Autodesk Fusion 360 part; units mm, degrees
(part 3 of 12)
  arc A1088 (217.4364, 35.2653) -> (218.9364, 35.2653) centre (218.1864, 35.2653) ccw
  arc A1089 (218.9364, 35.2653) -> (217.4364, 35.2653) centre (218.1864, 35.2653) ccw
  arc A1090 (218.9364, 37.8053) -> (217.4364, 37.8053) centre (218.1864, 37.8053) ccw
  arc A1091 (217.4364, 37.8053) -> (218.9364, 37.8053) centre (218.1864, 37.8053) ccw
  arc A1092 (217.4364, 37.8053) -> (218.9364, 37.8053) centre (218.1864, 37.8053) ccw
  arc A1093 (218.9364, 37.8053) -> (217.4364, 37.8053) centre (218.1864, 37.8053) ccw
  arc A1094 (218.9364, 37.8053) -> (217.4364, 37.8053) centre (218.1864, 37.8053) ccw
  arc A1095 (217.4364, 37.8053) -> (218.9364, 37.8053) centre (218.1864, 37.8053) ccw
  arc A1096 (209.8164, 4.7852) -> (211.3164, 4.7852) centre (210.5664, 4.7852) ccw
  arc A1097 (211.3164, 4.7852) -> (209.8164, 4.7852) centre (210.5664, 4.7852) ccw
  arc A1098 (209.8164, 4.7852) -> (211.3164, 4.7852) centre (210.5664, 4.7852) ccw
  arc A1099 (211.3164, 4.7852) -> (209.8164, 4.7852) centre (210.5664, 4.7852) ccw
  arc A1100 (211.3164, 4.7852) -> (209.8164, 4.7852) centre (210.5664, 4.7852) ccw
  arc A1101 (209.8164, 4.7852) -> (211.3164, 4.7852) centre (210.5664, 4.7852) ccw
  arc A1102 (209.8164, 7.3252) -> (211.3164, 7.3252) centre (210.5664, 7.3252) ccw
  arc A1103 (211.3164, 7.3252) -> (209.8164, 7.3252) centre (210.5664, 7.3252) ccw
  arc A1104 (209.8164, 7.3252) -> (211.3164, 7.3252) centre (210.5664, 7.3252) ccw
  arc A1105 (211.3164, 7.3252) -> (209.8164, 7.3252) centre (210.5664, 7.3252) ccw
  arc A1106 (211.3164, 7.3252) -> (209.8164, 7.3252) centre (210.5664, 7.3252) ccw
  arc A1107 (209.8164, 7.3252) -> (211.3164, 7.3252) centre (210.5664, 7.3252) ccw
  arc A1108 (209.8164, 9.8652) -> (211.3164, 9.8652) centre (210.5664, 9.8652) ccw
  arc A1109 (211.3164, 9.8652) -> (209.8164, 9.8652) centre (210.5664, 9.8652) ccw
  arc A1110 (209.8164, 9.8652) -> (211.3164, 9.8652) centre (210.5664, 9.8652) ccw
  arc A1111 (211.3164, 9.8652) -> (209.8164, 9.8652) centre (210.5664, 9.8652) ccw
  arc A1112 (209.8164, 9.8652) -> (211.3164, 9.8652) centre (210.5664, 9.8652) ccw
  arc A1113 (211.3164, 9.8652) -> (209.8164, 9.8652) centre (210.5664, 9.8652) ccw
  arc A1114 (211.3164, 12.4052) -> (209.8164, 12.4052) centre (210.5664, 12.4052) ccw
  arc A1115 (209.8164, 12.4052) -> (211.3164, 12.4052) centre (210.5664, 12.4052) ccw
  arc A1116 (211.3164, 12.4052) -> (209.8164, 12.4052) centre (210.5664, 12.4052) ccw
  arc A1117 (209.8164, 12.4052) -> (211.3164, 12.4052) centre (210.5664, 12.4052) ccw
  arc A1118 (209.8164, 12.4052) -> (211.3164, 12.4052) centre (210.5664, 12.4052) ccw
  arc A1119 (211.3164, 12.4052) -> (209.8164, 12.4052) centre (210.5664, 12.4052) ccw
  arc A1120 (211.3164, 14.9452) -> (209.8164, 14.9452) centre (210.5664, 14.9452) ccw
  arc A1121 (209.8164, 14.9452) -> (211.3164, 14.9452) centre (210.5664, 14.9452) ccw
  arc A1122 (209.8164, 14.9452) -> (211.3164, 14.9452) centre (210.5664, 14.9452) ccw
  arc A1123 (211.3164, 14.9452) -> (209.8164, 14.9452) centre (210.5664, 14.9452) ccw
  arc A1124 (211.3164, 14.9452) -> (209.8164, 14.9452) centre (210.5664, 14.9452) ccw
  arc A1125 (209.8164, 14.9452) -> (211.3164, 14.9452) centre (210.5664, 14.9452) ccw
  arc A1126 (209.8164, 17.4852) -> (211.3164, 17.4852) centre (210.5664, 17.4852) ccw
  arc A1127 (211.3164, 17.4852) -> (209.8164, 17.4852) centre (210.5664, 17.4852) ccw
  arc A1128 (209.8164, 17.4852) -> (211.3164, 17.4852) centre (210.5664, 17.4852) ccw
  arc A1129 (211.3164, 17.4852) -> (209.8164, 17.4852) centre (210.5664, 17.4852) ccw
  arc A1130 (211.3164, 17.4852) -> (209.8164, 17.4852) centre (210.5664, 17.4852) ccw
  arc A1131 (209.8164, 17.4852) -> (211.3164, 17.4852) centre (210.5664, 17.4852) ccw
  arc A1132 (211.3164, 20.0252) -> (209.8164, 20.0252) centre (210.5664, 20.0252) ccw
  arc A1133 (209.8164, 20.0252) -> (211.3164, 20.0252) centre (210.5664, 20.0252) ccw
  arc A1134 (209.8164, 20.0252) -> (211.3164, 20.0252) centre (210.5664, 20.0252) ccw
  arc A1135 (211.3164, 20.0252) -> (209.8164, 20.0252) centre (210.5664, 20.0252) ccw
  arc A1136 (209.8164, 20.0252) -> (211.3164, 20.0252) centre (210.5664, 20.0252) ccw
  arc A1137 (211.3164, 20.0252) -> (209.8164, 20.0252) centre (210.5664, 20.0252) ccw
  arc A1138 (209.8164, 22.5653) -> (211.3164, 22.5653) centre (210.5664, 22.5653) ccw
  arc A1139 (211.3164, 22.5653) -> (209.8164, 22.5653) centre (210.5664, 22.5653) ccw
  arc A1140 (209.8164, 22.5653) -> (211.3164, 22.5653) centre (210.5664, 22.5653) ccw
  arc A1141 (211.3164, 22.5653) -> (209.8164, 22.5653) centre (210.5664, 22.5653) ccw
  arc A1142 (209.8164, 22.5653) -> (211.3164, 22.5653) centre (210.5664, 22.5653) ccw
  arc A1143 (211.3164, 22.5653) -> (209.8164, 22.5653) centre (210.5664, 22.5653) ccw
  arc A1144 (211.3164, 25.1053) -> (209.8164, 25.1053) centre (210.5664, 25.1053) ccw
  arc A1145 (209.8164, 25.1053) -> (211.3164, 25.1053) centre (210.5664, 25.1053) ccw
  arc A1146 (209.8164, 25.1053) -> (211.3164, 25.1053) centre (210.5664, 25.1053) ccw
  arc A1147 (211.3164, 25.1053) -> (209.8164, 25.1053) centre (210.5664, 25.1053) ccw
  arc A1148 (211.3164, 25.1053) -> (209.8164, 25.1053) centre (210.5664, 25.1053) ccw
  arc A1149 (209.8164, 25.1053) -> (211.3164, 25.1053) centre (210.5664, 25.1053) ccw
  arc A1150 (211.3164, 27.6453) -> (209.8164, 27.6453) centre (210.5664, 27.6453) ccw
  arc A1151 (209.8164, 27.6453) -> (211.3164, 27.6453) centre (210.5664, 27.6453) ccw
  arc A1152 (211.3164, 27.6453) -> (209.8164, 27.6453) centre (210.5664, 27.6453) ccw
  arc A1153 (209.8164, 27.6453) -> (211.3164, 27.6453) centre (210.5664, 27.6453) ccw
  arc A1154 (211.3164, 27.6453) -> (209.8164, 27.6453) centre (210.5664, 27.6453) ccw
  arc A1155 (209.8164, 27.6453) -> (211.3164, 27.6453) centre (210.5664, 27.6453) ccw
  arc A1156 (209.8164, 30.1853) -> (211.3164, 30.1853) centre (210.5664, 30.1853) ccw
  arc A1157 (211.3164, 30.1853) -> (209.8164, 30.1853) centre (210.5664, 30.1853) ccw
  arc A1158 (211.3164, 30.1853) -> (209.8164, 30.1853) centre (210.5664, 30.1853) ccw
  arc A1159 (209.8164, 30.1853) -> (211.3164, 30.1853) centre (210.5664, 30.1853) ccw
  arc A1160 (211.3164, 30.1853) -> (209.8164, 30.1853) centre (210.5664, 30.1853) ccw
  arc A1161 (209.8164, 30.1853) -> (211.3164, 30.1853) centre (210.5664, 30.1853) ccw
  arc A1162 (211.3164, 32.7253) -> (209.8164, 32.7253) centre (210.5664, 32.7253) ccw
  arc A1163 (209.8164, 32.7253) -> (211.3164, 32.7253) centre (210.5664, 32.7253) ccw
  arc A1164 (211.3164, 32.7253) -> (209.8164, 32.7253) centre (210.5664, 32.7253) ccw
  arc A1165 (209.8164, 32.7253) -> (211.3164, 32.7253) centre (210.5664, 32.7253) ccw
  arc A1166 (209.8164, 32.7253) -> (211.3164, 32.7253) centre (210.5664, 32.7253) ccw
  arc A1167 (211.3164, 32.7253) -> (209.8164, 32.7253) centre (210.5664, 32.7253) ccw
  arc A1168 (211.3164, 35.2653) -> (209.8164, 35.2653) centre (210.5664, 35.2653) ccw
  arc A1169 (209.8164, 35.2653) -> (211.3164, 35.2653) centre (210.5664, 35.2653) ccw
  arc A1170 (209.8164, 35.2653) -> (211.3164, 35.2653) centre (210.5664, 35.2653) ccw
  arc A1171 (211.3164, 35.2653) -> (209.8164, 35.2653) centre (210.5664, 35.2653) ccw
  arc A1172 (209.8164, 35.2653) -> (211.3164, 35.2653) centre (210.5664, 35.2653) ccw
  arc A1173 (211.3164, 35.2653) -> (209.8164, 35.2653) centre (210.5664, 35.2653) ccw
  line L207 (211.3164, 38.5553) -> (211.3164, 37.0553)
  line L208 (211.3164, 37.0553) -> (209.8164, 37.0553)
  line L209 (209.8164, 38.5553) -> (211.3164, 38.5553)
  line L210 (209.8164, 37.0553) -> (209.8164, 38.5553)
  line L211 (209.8164, 38.5553) -> (211.3164, 38.5553)
  line L212 (211.3164, 37.0553) -> (209.8164, 37.0553)
  line L213 (211.3164, 38.5553) -> (211.3164, 37.0553)
  line L214 (209.8164, 37.0553) -> (209.8164, 38.5553)
  line L215 (211.3164, 37.0553) -> (209.8164, 37.0553)
  line L216 (209.8164, 38.5553) -> (211.3164, 38.5553)
  line L217 (211.3164, 38.5553) -> (211.3164, 37.0553)
  line L218 (209.8164, 37.0553) -> (209.8164, 38.5553)
  arc A1174 (129.4564, -32.864) -> (131.9964, -32.864) centre (130.7264, -32.864) ccw
  arc A1175 (131.9964, -32.864) -> (129.4564, -32.864) centre (130.7264, -32.864) ccw
  arc A1176 (129.4564, -32.864) -> (131.9964, -32.864) centre (130.7264, -32.864) ccw
  arc A1177 (131.9964, -32.864) -> (129.4564, -32.864) centre (130.7264, -32.864) ccw
  arc A1178 (131.9964, -32.864) -> (129.4564, -32.864) centre (130.7264, -32.864) ccw
  arc A1179 (129.4564, -32.864) -> (131.9964, -32.864) centre (130.7264, -32.864) ccw
  arc A1180 (123.1064, -35.404) -> (125.6464, -35.404) centre (124.3764, -35.404) ccw
  arc A1181 (125.6464, -35.404) -> (123.1064, -35.404) centre (124.3764, -35.404) ccw
  arc A1182 (123.1064, -35.404) -> (125.6464, -35.404) centre (124.3764, -35.404) ccw
  arc A1183 (125.6464, -35.404) -> (123.1064, -35.404) centre (124.3764, -35.404) ccw
  arc A1184 (125.6464, -35.404) -> (123.1064, -35.404) centre (124.3764, -35.404) ccw
  arc A1185 (123.1064, -35.404) -> (125.6464, -35.404) centre (124.3764, -35.404) ccw
  arc A1186 (161.9964, -32.864) -> (159.4564, -32.864) centre (160.7264, -32.864) ccw
  arc A1187 (159.4564, -32.864) -> (161.9964, -32.864) centre (160.7264, -32.864) ccw
  arc A1188 (161.9964, -32.864) -> (159.4564, -32.864) centre (160.7264, -32.864) ccw
  arc A1189 (159.4564, -32.864) -> (161.9964, -32.864) centre (160.7264, -32.864) ccw
  arc A1190 (159.4564, -32.864) -> (161.9964, -32.864) centre (160.7264, -32.864) ccw
  arc A1191 (161.9964, -32.864) -> (159.4564, -32.864) centre (160.7264, -32.864) ccw
  arc A1192 (153.1064, -35.404) -> (155.6464, -35.404) centre (154.3764, -35.404) ccw
  arc A1193 (155.6464, -35.404) -> (153.1064, -35.404) centre (154.3764, -35.404) ccw
  arc A1194 (153.1064, -35.404) -> (155.6464, -35.404) centre (154.3764, -35.404) ccw
  arc A1195 (155.6464, -35.404) -> (153.1064, -35.404) centre (154.3764, -35.404) ccw
  arc A1196 (155.6464, -35.404) -> (153.1064, -35.404) centre (154.3764, -35.404) ccw
  arc A1197 (153.1064, -35.404) -> (155.6464, -35.404) centre (154.3764, -35.404) ccw
  arc A1198 (189.4564, -32.864) -> (191.9964, -32.864) centre (190.7264, -32.864) ccw
  arc A1199 (191.9964, -32.864) -> (189.4564, -32.864) centre (190.7264, -32.864) ccw
  arc A1200 (191.9964, -32.864) -> (189.4564, -32.864) centre (190.7264, -32.864) ccw
  arc A1201 (189.4564, -32.864) -> (191.9964, -32.864) centre (190.7264, -32.864) ccw
  arc A1202 (189.4564, -32.864) -> (191.9964, -32.864) centre (190.7264, -32.864) ccw
  arc A1203 (191.9964, -32.864) -> (189.4564, -32.864) centre (190.7264, -32.864) ccw
  arc A1204 (185.6464, -35.404) -> (183.1064, -35.404) centre (184.3764, -35.404) ccw
  arc A1205 (183.1064, -35.404) -> (185.6464, -35.404) centre (184.3764, -35.404) ccw
  arc A1206 (185.6464, -35.404) -> (183.1064, -35.404) centre (184.3764, -35.404) ccw
  arc A1207 (183.1064, -35.404) -> (185.6464, -35.404) centre (184.3764, -35.404) ccw
  arc A1208 (183.1064, -35.404) -> (185.6464, -35.404) centre (184.3764, -35.404) ccw
  arc A1209 (185.6464, -35.404) -> (183.1064, -35.404) centre (184.3764, -35.404) ccw
  arc A1210 (219.4564, -32.864) -> (221.9964, -32.864) centre (220.7264, -32.864) ccw
  arc A1211 (221.9964, -32.864) -> (219.4564, -32.864) centre (220.7264, -32.864) ccw
  arc A1212 (219.4564, -32.864) -> (221.9964, -32.864) centre (220.7264, -32.864) ccw
  arc A1213 (221.9964, -32.864) -> (219.4564, -32.864) centre (220.7264, -32.864) ccw
  arc A1214 (221.9964, -32.864) -> (219.4564, -32.864) centre (220.7264, -32.864) ccw
  arc A1215 (219.4564, -32.864) -> (221.9964, -32.864) centre (220.7264, -32.864) ccw
  arc A1216 (213.1064, -35.404) -> (215.6464, -35.404) centre (214.3764, -35.404) ccw
  arc A1217 (215.6464, -35.404) -> (213.1064, -35.404) centre (214.3764, -35.404) ccw
  arc A1218 (213.1064, -35.404) -> (215.6464, -35.404) centre (214.3764, -35.404) ccw
  arc A1219 (215.6464, -35.404) -> (213.1064, -35.404) centre (214.3764, -35.404) ccw
  arc A1220 (213.1064, -35.404) -> (215.6464, -35.404) centre (214.3764, -35.404) ccw
  arc A1221 (215.6464, -35.404) -> (213.1064, -35.404) centre (214.3764, -35.404) ccw
  arc A1222 (208.7884, -60.2389) -> (206.2484, -60.2389) centre (207.5184, -60.2389) ccw
  arc A1223 (206.2484, -60.2389) -> (208.7884, -60.2389) centre (207.5184, -60.2389) ccw
  arc A1224 (208.7884, -60.2389) -> (206.2484, -60.2389) centre (207.5184, -60.2389) ccw
  arc A1225 (206.2484, -60.2389) -> (208.7884, -60.2389) centre (207.5184, -60.2389) ccw
  arc A1226 (206.2484, -60.2389) -> (208.7884, -60.2389) centre (207.5184, -60.2389) ccw
  arc A1227 (208.7884, -60.2389) -> (206.2484, -60.2389) centre (207.5184, -60.2389) ccw
  arc A1228 (202.4384, -62.7789) -> (199.8984, -62.7789) centre (201.1684, -62.7789) ccw
  arc A1229 (199.8984, -62.7789) -> (202.4384, -62.7789) centre (201.1684, -62.7789) ccw
  arc A1230 (202.4384, -62.7789) -> (199.8984, -62.7789) centre (201.1684, -62.7789) ccw
  arc A1231 (199.8984, -62.7789) -> (202.4384, -62.7789) centre (201.1684, -62.7789) ccw
  arc A1232 (202.4384, -62.7789) -> (199.8984, -62.7789) centre (201.1684, -62.7789) ccw
  arc A1233 (199.8984, -62.7789) -> (202.4384, -62.7789) centre (201.1684, -62.7789) ccw
  arc A1234 (42.9261, -60.2389) -> (45.4661, -60.2389) centre (44.1961, -60.2389) ccw
  arc A1235 (45.4661, -60.2389) -> (42.9261, -60.2389) centre (44.1961, -60.2389) ccw
  arc A1236 (45.4661, -60.2389) -> (42.9261, -60.2389) centre (44.1961, -60.2389) ccw
  arc A1237 (42.9261, -60.2389) -> (45.4661, -60.2389) centre (44.1961, -60.2389) ccw
  arc A1238 (45.4661, -60.2389) -> (42.9261, -60.2389) centre (44.1961, -60.2389) ccw
  arc A1239 (42.9261, -60.2389) -> (45.4661, -60.2389) centre (44.1961, -60.2389) ccw
  arc A1240 (39.1161, -62.7789) -> (36.5761, -62.7789) centre (37.8461, -62.7789) ccw
  arc A1241 (36.5761, -62.7789) -> (39.1161, -62.7789) centre (37.8461, -62.7789) ccw
  arc A1242 (36.5761, -62.7789) -> (39.1161, -62.7789) centre (37.8461, -62.7789) ccw
  arc A1243 (39.1161, -62.7789) -> (36.5761, -62.7789) centre (37.8461, -62.7789) ccw
  arc A1244 (36.5761, -62.7789) -> (39.1161, -62.7789) centre (37.8461, -62.7789) ccw
  arc A1245 (39.1161, -62.7789) -> (36.5761, -62.7789) centre (37.8461, -62.7789) ccw
  arc A1246 (79.6292, -60.2389) -> (77.0892, -60.2389) centre (78.3592, -60.2389) ccw
  arc A1247 (77.0892, -60.2389) -> (79.6292, -60.2389) centre (78.3592, -60.2389) ccw
  arc A1248 (77.0892, -60.2389) -> (79.6292, -60.2389) centre (78.3592, -60.2389) ccw
  arc A1249 (79.6292, -60.2389) -> (77.0892, -60.2389) centre (78.3592, -60.2389) ccw
  arc A1250 (79.6292, -60.2389) -> (77.0892, -60.2389) centre (78.3592, -60.2389) ccw
  arc A1251 (77.0892, -60.2389) -> (79.6292, -60.2389) centre (78.3592, -60.2389) ccw
  arc A1252 (70.7391, -62.7789) -> (73.2791, -62.7789) centre (72.0091, -62.7789) ccw
  arc A1253 (73.2791, -62.7789) -> (70.7391, -62.7789) centre (72.0091, -62.7789) ccw
  arc A1254 (70.7391, -62.7789) -> (73.2791, -62.7789) centre (72.0091, -62.7789) ccw
  arc A1255 (73.2791, -62.7789) -> (70.7391, -62.7789) centre (72.0091, -62.7789) ccw
  arc A1256 (70.7391, -62.7789) -> (73.2791, -62.7789) centre (72.0091, -62.7789) ccw
  arc A1257 (73.2791, -62.7789) -> (70.7391, -62.7789) centre (72.0091, -62.7789) ccw
  arc A1258 (18.022, -2.3268) -> (16.522, -2.3268) centre (17.272, -2.3268) ccw
  arc A1259 (16.522, -2.3268) -> (18.022, -2.3268) centre (17.272, -2.3268) ccw
  arc A1260 (16.522, -2.3268) -> (18.022, -2.3268) centre (17.272, -2.3268) ccw
  arc A1261 (18.022, -2.3268) -> (16.522, -2.3268) centre (17.272, -2.3268) ccw
  arc A1262 (18.022, -2.3268) -> (16.522, -2.3268) centre (17.272, -2.3268) ccw
  arc A1263 (16.522, -2.3268) -> (18.022, -2.3268) centre (17.272, -2.3268) ccw
  arc A1264 (18.022, 0.2132) -> (16.522, 0.2132) centre (17.272, 0.2132) ccw
  arc A1265 (16.522, 0.2132) -> (18.022, 0.2132) centre (17.272, 0.2132) ccw
  arc A1266 (16.522, 0.2132) -> (18.022, 0.2132) centre (17.272, 0.2132) ccw
  arc A1267 (18.022, 0.2132) -> (16.522, 0.2132) centre (17.272, 0.2132) ccw
  arc A1268 (16.522, 0.2132) -> (18.022, 0.2132) centre (17.272, 0.2132) ccw
  arc A1269 (18.022, 0.2132) -> (16.522, 0.2132) centre (17.272, 0.2132) ccw
  arc A1270 (16.522, 2.7532) -> (18.022, 2.7532) centre (17.272, 2.7532) ccw
  arc A1271 (18.022, 2.7532) -> (16.522, 2.7532) centre (17.272, 2.7532) ccw
  arc A1272 (16.522, 2.7532) -> (18.022, 2.7532) centre (17.272, 2.7532) ccw
  arc A1273 (18.022, 2.7532) -> (16.522, 2.7532) centre (17.272, 2.7532) ccw
  arc A1274 (16.522, 2.7532) -> (18.022, 2.7532) centre (17.272, 2.7532) ccw
  arc A1275 (18.022, 2.7532) -> (16.522, 2.7532) centre (17.272, 2.7532) ccw
  arc A1276 (18.022, 5.2932) -> (16.522, 5.2932) centre (17.272, 5.2932) ccw
  arc A1277 (16.522, 5.2932) -> (18.022, 5.2932) centre (17.272, 5.2932) ccw
  arc A1278 (18.022, 5.2932) -> (16.522, 5.2932) centre (17.272, 5.2932) ccw
  arc A1279 (16.522, 5.2932) -> (18.022, 5.2932) centre (17.272, 5.2932) ccw
  arc A1280 (18.022, 5.2932) -> (16.522, 5.2932) centre (17.272, 5.2932) ccw
  arc A1281 (16.522, 5.2932) -> (18.022, 5.2932) centre (17.272, 5.2932) ccw
  arc A1282 (18.022, 7.8332) -> (16.522, 7.8332) centre (17.272, 7.8332) ccw
  arc A1283 (16.522, 7.8332) -> (18.022, 7.8332) centre (17.272, 7.8332) ccw
  arc A1284 (16.522, 7.8332) -> (18.022, 7.8332) centre (17.272, 7.8332) ccw
  arc A1285 (18.022, 7.8332) -> (16.522, 7.8332) centre (17.272, 7.8332) ccw
  arc A1286 (16.522, 7.8332) -> (18.022, 7.8332) centre (17.272, 7.8332) ccw
  arc A1287 (18.022, 7.8332) -> (16.522, 7.8332) centre (17.272, 7.8332) ccw
  arc A1288 (16.522, 10.3732) -> (18.022, 10.3732) centre (17.272, 10.3732) ccw
  arc A1289 (18.022, 10.3732) -> (16.522, 10.3732) centre (17.272, 10.3732) ccw
  arc A1290 (16.522, 10.3732) -> (18.022, 10.3732) centre (17.272, 10.3732) ccw
  arc A1291 (18.022, 10.3732) -> (16.522, 10.3732) centre (17.272, 10.3732) ccw
  arc A1292 (18.022, 10.3732) -> (16.522, 10.3732) centre (17.272, 10.3732) ccw
  arc A1293 (16.522, 10.3732) -> (18.022, 10.3732) centre (17.272, 10.3732) ccw
  arc A1294 (16.522, 12.9132) -> (18.022, 12.9132) centre (17.272, 12.9132) ccw
  arc A1295 (18.022, 12.9132) -> (16.522, 12.9132) centre (17.272, 12.9132) ccw
  arc A1296 (16.522, 12.9132) -> (18.022, 12.9132) centre (17.272, 12.9132) ccw
  arc A1297 (18.022, 12.9132) -> (16.522, 12.9132) centre (17.272, 12.9132) ccw
  arc A1298 (16.522, 12.9132) -> (18.022, 12.9132) centre (17.272, 12.9132) ccw
  arc A1299 (18.022, 12.9132) -> (16.522, 12.9132) centre (17.272, 12.9132) ccw
  arc A1300 (16.522, 15.4532) -> (18.022, 15.4532) centre (17.272, 15.4532) ccw
  arc A1301 (18.022, 15.4532) -> (16.522, 15.4532) centre (17.272, 15.4532) ccw
  arc A1302 (16.522, 15.4532) -> (18.022, 15.4532) centre (17.272, 15.4532) ccw
  arc A1303 (18.022, 15.4532) -> (16.522, 15.4532) centre (17.272, 15.4532) ccw
  arc A1304 (16.522, 15.4532) -> (18.022, 15.4532) centre (17.272, 15.4532) ccw
  arc A1305 (18.022, 15.4532) -> (16.522, 15.4532) centre (17.272, 15.4532) ccw
  arc A1306 (16.522, 17.9932) -> (18.022, 17.9932) centre (17.272, 17.9932) ccw
  arc A1307 (18.022, 17.9932) -> (16.522, 17.9932) centre (17.272, 17.9932) ccw
  arc A1308 (16.522, 17.9932) -> (18.022, 17.9932) centre (17.272, 17.9932) ccw
  arc A1309 (18.022, 17.9932) -> (16.522, 17.9932) centre (17.272, 17.9932) ccw
  arc A1310 (16.522, 17.9932) -> (18.022, 17.9932) centre (17.272, 17.9932) ccw
  arc A1311 (18.022, 17.9932) -> (16.522, 17.9932) centre (17.272, 17.9932) ccw
  arc A1312 (18.022, 20.5332) -> (16.522, 20.5332) centre (17.272, 20.5332) ccw
  arc A1313 (16.522, 20.5332) -> (18.022, 20.5332) centre (17.272, 20.5332) ccw
  arc A1314 (18.022, 20.5332) -> (16.522, 20.5332) centre (17.272, 20.5332) ccw
  arc A1315 (16.522, 20.5332) -> (18.022, 20.5332) centre (17.272, 20.5332) ccw
  arc A1316 (16.522, 20.5332) -> (18.022, 20.5332) centre (17.272, 20.5332) ccw
  arc A1317 (18.022, 20.5332) -> (16.522, 20.5332) centre (17.272, 20.5332) ccw
  arc A1318 (16.522, 23.0733) -> (18.022, 23.0733) centre (17.272, 23.0733) ccw
  arc A1319 (18.022, 23.0733) -> (16.522, 23.0733) centre (17.272, 23.0733) ccw
  arc A1320 (16.522, 23.0733) -> (18.022, 23.0733) centre (17.272, 23.0733) ccw
  arc A1321 (18.022, 23.0733) -> (16.522, 23.0733) centre (17.272, 23.0733) ccw
  arc A1322 (16.522, 23.0733) -> (18.022, 23.0733) centre (17.272, 23.0733) ccw
  arc A1323 (18.022, 23.0733) -> (16.522, 23.0733) centre (17.272, 23.0733) ccw
  arc A1324 (16.522, 25.6133) -> (18.022, 25.6133) centre (17.272, 25.6133) ccw
  arc A1325 (18.022, 25.6133) -> (16.522, 25.6133) centre (17.272, 25.6133) ccw
  arc A1326 (16.522, 25.6133) -> (18.022, 25.6133) centre (17.272, 25.6133) ccw
  arc A1327 (18.022, 25.6133) -> (16.522, 25.6133) centre (17.272, 25.6133) ccw
  arc A1328 (16.522, 25.6133) -> (18.022, 25.6133) centre (17.272, 25.6133) ccw
  arc A1329 (18.022, 25.6133) -> (16.522, 25.6133) centre (17.272, 25.6133) ccw
  arc A1330 (16.522, 28.1533) -> (18.022, 28.1533) centre (17.272, 28.1533) ccw
  arc A1331 (18.022, 28.1533) -> (16.522, 28.1533) centre (17.272, 28.1533) ccw
  arc A1332 (16.522, 28.1533) -> (18.022, 28.1533) centre (17.272, 28.1533) ccw
  arc A1333 (18.022, 28.1533) -> (16.522, 28.1533) centre (17.272, 28.1533) ccw
  arc A1334 (16.522, 28.1533) -> (18.022, 28.1533) centre (17.272, 28.1533) ccw
  arc A1335 (18.022, 28.1533) -> (16.522, 28.1533) centre (17.272, 28.1533) ccw
  arc A1336 (16.522, 30.6933) -> (18.022, 30.6933) centre (17.272, 30.6933) ccw
  arc A1337 (18.022, 30.6933) -> (16.522, 30.6933) centre (17.272, 30.6933) ccw
  arc A1338 (16.522, 30.6933) -> (18.022, 30.6933) centre (17.272, 30.6933) ccw
  arc A1339 (18.022, 30.6933) -> (16.522, 30.6933) centre (17.272, 30.6933) ccw
  arc A1340 (16.522, 30.6933) -> (18.022, 30.6933) centre (17.272, 30.6933) ccw
  arc A1341 (18.022, 30.6933) -> (16.522, 30.6933) centre (17.272, 30.6933) ccw
  arc A1342 (8.902, -2.3268) -> (10.402, -2.3268) centre (9.652, -2.3268) ccw
  arc A1343 (10.402, -2.3268) -> (8.902, -2.3268) centre (9.652, -2.3268) ccw
  arc A1344 (8.902, -2.3268) -> (10.402, -2.3268) centre (9.652, -2.3268) ccw
  arc A1345 (10.402, -2.3268) -> (8.902, -2.3268) centre (9.652, -2.3268) ccw
  arc A1346 (8.902, -2.3268) -> (10.402, -2.3268) centre (9.652, -2.3268) ccw
  arc A1347 (10.402, -2.3268) -> (8.902, -2.3268) centre (9.652, -2.3268) ccw
  arc A1348 (10.402, 0.2132) -> (8.902, 0.2132) centre (9.652, 0.2132) ccw
  arc A1349 (8.902, 0.2132) -> (10.402, 0.2132) centre (9.652, 0.2132) ccw
  arc A1350 (10.402, 0.2132) -> (8.902, 0.2132) centre (9.652, 0.2132) ccw
  arc A1351 (8.902, 0.2132) -> (10.402, 0.2132) centre (9.652, 0.2132) ccw
  arc A1352 (8.902, 0.2132) -> (10.402, 0.2132) centre (9.652, 0.2132) ccw
  arc A1353 (10.402, 0.2132) -> (8.902, 0.2132) centre (9.652, 0.2132) ccw
  arc A1354 (8.902, 2.7532) -> (10.402, 2.7532) centre (9.652, 2.7532) ccw
  arc A1355 (10.402, 2.7532) -> (8.902, 2.7532) centre (9.652, 2.7532) ccw
  arc A1356 (8.902, 2.7532) -> (10.402, 2.7532) centre (9.652, 2.7532) ccw
  arc A1357 (10.402, 2.7532) -> (8.902, 2.7532) centre (9.652, 2.7532) ccw
  arc A1358 (8.902, 2.7532) -> (10.402, 2.7532) centre (9.652, 2.7532) ccw
  arc A1359 (10.402, 2.7532) -> (8.902, 2.7532) centre (9.652, 2.7532) ccw
  arc A1360 (8.902, 5.2932) -> (10.402, 5.2932) centre (9.652, 5.2932) ccw
  arc A1361 (10.402, 5.2932) -> (8.902, 5.2932) centre (9.652, 5.2932) ccw
  arc A1362 (8.902, 5.2932) -> (10.402, 5.2932) centre (9.652, 5.2932) ccw
  arc A1363 (10.402, 5.2932) -> (8.902, 5.2932) centre (9.652, 5.2932) ccw
  arc A1364 (8.902, 5.2932) -> (10.402, 5.2932) centre (9.652, 5.2932) ccw
  arc A1365 (10.402, 5.2932) -> (8.902, 5.2932) centre (9.652, 5.2932) ccw
  arc A1366 (10.402, 7.8332) -> (8.902, 7.8332) centre (9.652, 7.8332) ccw
  arc A1367 (8.902, 7.8332) -> (10.402, 7.8332) centre (9.652, 7.8332) ccw
  arc A1368 (10.402, 7.8332) -> (8.902, 7.8332) centre (9.652, 7.8332) ccw
  arc A1369 (8.902, 7.8332) -> (10.402, 7.8332) centre (9.652, 7.8332) ccw
  arc A1370 (10.402, 7.8332) -> (8.902, 7.8332) centre (9.652, 7.8332) ccw
  arc A1371 (8.902, 7.8332) -> (10.402, 7.8332) centre (9.652, 7.8332) ccw
  arc A1372 (10.402, 10.3732) -> (8.902, 10.3732) centre (9.652, 10.3732) ccw
  arc A1373 (8.902, 10.3732) -> (10.402, 10.3732) centre (9.652, 10.3732) ccw
  arc A1374 (8.902, 10.3732) -> (10.402, 10.3732) centre (9.652, 10.3732) ccw
  arc A1375 (10.402, 10.3732) -> (8.902, 10.3732) centre (9.652, 10.3732) ccw
  arc A1376 (8.902, 10.3732) -> (10.402, 10.3732) centre (9.652, 10.3732) ccw
  arc A1377 (10.402, 10.3732) -> (8.902, 10.3732) centre (9.652, 10.3732) ccw
  arc A1378 (8.902, 12.9132) -> (10.402, 12.9132) centre (9.652, 12.9132) ccw
  arc A1379 (10.402, 12.9132) -> (8.902, 12.9132) centre (9.652, 12.9132) ccw
  arc A1380 (8.902, 12.9132) -> (10.402, 12.9132) centre (9.652, 12.9132) ccw
  arc A1381 (10.402, 12.9132) -> (8.902, 12.9132) centre (9.652, 12.9132) ccw
  arc A1382 (8.902, 12.9132) -> (10.402, 12.9132) centre (9.652, 12.9132) ccw
  arc A1383 (10.402, 12.9132) -> (8.902, 12.9132) centre (9.652, 12.9132) ccw
  arc A1384 (8.902, 15.4532) -> (10.402, 15.4532) centre (9.652, 15.4532) ccw
  arc A1385 (10.402, 15.4532) -> (8.902, 15.4532) centre (9.652, 15.4532) ccw
  arc A1386 (8.902, 15.4532) -> (10.402, 15.4532) centre (9.652, 15.4532) ccw
  arc A1387 (10.402, 15.4532) -> (8.902, 15.4532) centre (9.652, 15.4532) ccw
  arc A1388 (10.402, 15.4532) -> (8.902, 15.4532) centre (9.652, 15.4532) ccw
  arc A1389 (8.902, 15.4532) -> (10.402, 15.4532) centre (9.652, 15.4532) ccw
  arc A1390 (8.902, 17.9932) -> (10.402, 17.9932) centre (9.652, 17.9932) ccw
  arc A1391 (10.402, 17.9932) -> (8.902, 17.9932) centre (9.652, 17.9932) ccw
  arc A1392 (8.902, 17.9932) -> (10.402, 17.9932) centre (9.652, 17.9932) ccw
  arc A1393 (10.402, 17.9932) -> (8.902, 17.9932) centre (9.652, 17.9932) ccw
  arc A1394 (8.902, 17.9932) -> (10.402, 17.9932) centre (9.652, 17.9932) ccw
  arc A1395 (10.402, 17.9932) -> (8.902, 17.9932) centre (9.652, 17.9932) ccw
  arc A1396 (8.902, 20.5332) -> (10.402, 20.5332) centre (9.652, 20.5332) ccw
  arc A1397 (10.402, 20.5332) -> (8.902, 20.5332) centre (9.652, 20.5332) ccw
  arc A1398 (8.902, 20.5332) -> (10.402, 20.5332) centre (9.652, 20.5332) ccw
  arc A1399 (10.402, 20.5332) -> (8.902, 20.5332) centre (9.652, 20.5332) ccw
  arc A1400 (8.902, 20.5332) -> (10.402, 20.5332) centre (9.652, 20.5332) ccw
  arc A1401 (10.402, 20.5332) -> (8.902, 20.5332) centre (9.652, 20.5332) ccw
  arc A1402 (8.902, 23.0733) -> (10.402, 23.0733) centre (9.652, 23.0733) ccw
  arc A1403 (10.402, 23.0733) -> (8.902, 23.0733) centre (9.652, 23.0733) ccw
  arc A1404 (8.902, 23.0733) -> (10.402, 23.0733) centre (9.652, 23.0733) ccw
  arc A1405 (10.402, 23.0733) -> (8.902, 23.0733) centre (9.652, 23.0733) ccw
  arc A1406 (8.902, 23.0733) -> (10.402, 23.0733) centre (9.652, 23.0733) ccw
  arc A1407 (10.402, 23.0733) -> (8.902, 23.0733) centre (9.652, 23.0733) ccw
  arc A1408 (10.402, 25.6133) -> (8.902, 25.6133) centre (9.652, 25.6133) ccw
  arc A1409 (8.902, 25.6133) -> (10.402, 25.6133) centre (9.652, 25.6133) ccw
  arc A1410 (8.902, 25.6133) -> (10.402, 25.6133) centre (9.652, 25.6133) ccw
  arc A1411 (10.402, 25.6133) -> (8.902, 25.6133) centre (9.652, 25.6133) ccw
  arc A1412 (8.902, 25.6133) -> (10.402, 25.6133) centre (9.652, 25.6133) ccw
  arc A1413 (10.402, 25.6133) -> (8.902, 25.6133) centre (9.652, 25.6133) ccw
  arc A1414 (8.902, 28.1533) -> (10.402, 28.1533) centre (9.652, 28.1533) ccw
  arc A1415 (10.402, 28.1533) -> (8.902, 28.1533) centre (9.652, 28.1533) ccw
  arc A1416 (8.902, 28.1533) -> (10.402, 28.1533) centre (9.652, 28.1533) ccw
  arc A1417 (10.402, 28.1533) -> (8.902, 28.1533) centre (9.652, 28.1533) ccw
  arc A1418 (10.402, 28.1533) -> (8.902, 28.1533) centre (9.652, 28.1533) ccw
  arc A1419 (8.902, 28.1533) -> (10.402, 28.1533) centre (9.652, 28.1533) ccw
  line L219 (10.402, 31.4433) -> (10.402, 29.9433)
  line L220 (8.902, 29.9433) -> (8.902, 31.4433)
  line L221 (8.902, 31.4433) -> (10.402, 31.4433)
  line L222 (10.402, 29.9433) -> (8.902, 29.9433)
  line L223 (10.402, 29.9433) -> (8.902, 29.9433)
  line L224 (10.402, 31.4433) -> (10.402, 29.9433)
  line L225 (8.902, 31.4433) -> (10.402, 31.4433)
  line L226 (8.902, 29.9433) -> (8.902, 31.4433)
  line L227 (10.402, 31.4433) -> (10.402, 29.9433)
  line L228 (8.902, 31.4433) -> (10.402, 31.4433)
  line L229 (8.902, 29.9433) -> (8.902, 31.4433)
  line L230 (10.402, 29.9433) -> (8.902, 29.9433)
  line L231 (208.3381, 77.3686) -> (208.3381, 79.8686)
  line L232 (208.3381, 79.8686) -> (209.8381, 79.8686)
  line L233 (209.8381, 79.8686) -> (209.8381, 77.3686)
  line L234 (209.8381, 77.3686) -> (208.3381, 77.3686)
  line L235 (209.8381, 79.8686) -> (209.8381, 77.3686)
  line L236 (208.3381, 77.3686) -> (208.3381, 79.8686)
  line L237 (208.3381, 79.8686) -> (209.8381, 79.8686)
  line L238 (209.8381, 77.3686) -> (208.3381, 77.3686)
  line L239 (209.8381, 77.3686) -> (208.3381, 77.3686)
  line L240 (209.8381, 79.8686) -> (209.8381, 77.3686)
  line L241 (208.3381, 79.8686) -> (209.8381, 79.8686)
  line L242 (208.3381, 77.3686) -> (208.3381, 79.8686)
  line L243 (203.9287, 78.8688) -> (205.4287, 78.8688)
  line L244 (203.9287, 76.3688) -> (203.9287, 78.8688)
  line L245 (205.4287, 76.3688) -> (203.9287, 76.3688)
  line L246 (205.4287, 78.8688) -> (205.4287, 76.3688)
  line L247 (205.4287, 76.3688) -> (203.9287, 76.3688)
  line L248 (205.4287, 78.8688) -> (205.4287, 76.3688)
  line L249 (203.9287, 78.8688) -> (205.4287, 78.8688)
  line L250 (203.9287, 76.3688) -> (203.9287, 78.8688)
  line L251 (205.4287, 76.3688) -> (203.9287, 76.3688)
  line L252 (205.4287, 78.8688) -> (205.4287, 76.3688)
  line L253 (203.9287, 78.8688) -> (205.4287, 78.8688)
  line L254 (203.9287, 76.3688) -> (203.9287, 78.8688)
  line L255 (209.8381, 81.3686) -> (208.3381, 81.3686)
  line L256 (209.8381, 83.8686) -> (209.8381, 81.3686)
  line L257 (208.3381, 83.8686) -> (209.8381, 83.8686)
  line L258 (208.3381, 81.3686) -> (208.3381, 83.8686)
  line L259 (208.3381, 83.8686) -> (209.8381, 83.8686)
  line L260 (208.3381, 81.3686) -> (208.3381, 83.8686)
  line L261 (209.8381, 81.3686) -> (208.3381, 81.3686)
  line L262 (209.8381, 83.8686) -> (209.8381, 81.3686)
  line L263 (208.3381, 81.3686) -> (208.3381, 83.8686)
  line L264 (208.3381, 83.8686) -> (209.8381, 83.8686)
  line L265 (209.8381, 83.8686) -> (209.8381, 81.3686)
  line L266 (209.8381, 81.3686) -> (208.3381, 81.3686)
  line L267 (209.8381, 87.2077) -> (209.8381, 84.7077)
  line L268 (208.3381, 84.7077) -> (208.3381, 87.2077)
  line L269 (209.8381, 84.7077) -> (208.3381, 84.7077)
  line L270 (208.3381, 87.2077) -> (209.8381, 87.2077)
  line L271 (209.8381, 84.7077) -> (208.3381, 84.7077)
  line L272 (209.8381, 87.2077) -> (209.8381, 84.7077)
  line L273 (208.3381, 87.2077) -> (209.8381, 87.2077)
  line L274 (208.3381, 84.7077) -> (208.3381, 87.2077)
  line L275 (209.8381, 84.7077) -> (208.3381, 84.7077)
  line L276 (209.8381, 87.2077) -> (209.8381, 84.7077)
  line L277 (208.3381, 87.2077) -> (209.8381, 87.2077)
  line L278 (208.3381, 84.7077) -> (208.3381, 87.2077)
  arc A1420 (15.7643, -58.0817) -> (16.3743, -58.0817) centre (16.0693, -58.0817) ccw
  arc A1421 (16.3743, -58.0817) -> (15.7643, -58.0817) centre (16.0693, -58.0817) ccw
  arc A1422 (8.917, -32.9778) -> (9.527, -32.9778) centre (9.222, -32.9778) ccw
  arc A1423 (9.527, -32.9778) -> (8.917, -32.9778) centre (9.222, -32.9778) ccw
  arc A1424 (211.917, 39.9996) -> (212.527, 39.9996) centre (212.222, 39.9996) ccw
  arc A1425 (212.527, 39.9996) -> (211.917, 39.9996) centre (212.222, 39.9996) ccw
  arc A1426 (38.4943, -70.5666) -> (39.1043, -70.5666) centre (38.7993, -70.5666) ccw
  arc A1427 (39.1043, -70.5666) -> (38.4943, -70.5666) centre (38.7993, -70.5666) ccw
  arc A1428 (79.5677, -71.3265) -> (80.1777, -71.3265) centre (79.8727, -71.3265) ccw
  arc A1429 (80.1777, -71.3265) -> (79.5677, -71.3265) centre (79.8727, -71.3265) ccw
  arc A1430 (73.3163, -54.9445) -> (73.9263, -54.9445) centre (73.6213, -54.9445) ccw
  arc A1431 (73.9263, -54.9445) -> (73.3163, -54.9445) centre (73.6213, -54.9445) ccw
  arc A1432 (198.4532, -67.6341) -> (199.0632, -67.6341) centre (198.7582, -67.6341) ccw
  arc A1433 (199.0632, -67.6341) -> (198.4532, -67.6341) centre (198.7582, -67.6341) ccw
  arc A1434 (46.6848, -67.6341) -> (47.2948, -67.6341) centre (46.9898, -67.6341) ccw
  arc A1435 (47.2948, -67.6341) -> (46.6848, -67.6341) centre (46.9898, -67.6341) ccw
  arc A1436 (216.4956, 25.5439) -> (217.1056, 25.5439) centre (216.8006, 25.5439) ccw
  arc A1437 (217.1056, 25.5439) -> (216.4956, 25.5439) centre (216.8006, 25.5439) ccw
  arc A1438 (40.4524, -31.2036) -> (41.0624, -31.2036) centre (40.7574, -31.2036) ccw
  arc A1439 (41.0624, -31.2036) -> (40.4524, -31.2036) centre (40.7574, -31.2036) ccw
  arc A1440 (18.3694, 22.7108) -> (18.9794, 22.7108) centre (18.6744, 22.7108) ccw
  arc A1441 (18.9794, 22.7108) -> (18.3694, 22.7108) centre (18.6744, 22.7108) ccw
  arc A1442 (155.8745, -41.9994) -> (155.2645, -41.9994) centre (155.5695, -41.9994) ccw
  arc A1443 (155.2645, -41.9994) -> (155.8745, -41.9994) centre (155.5695, -41.9994) ccw
  arc A1444 (190.4475, -40.1378) -> (189.8375, -40.1378) centre (190.1425, -40.1378) ccw
  arc A1445 (189.8375, -40.1378) -> (190.4475, -40.1378) centre (190.1425, -40.1378) ccw
  arc A1446 (125.2246, -43.2072) -> (125.8346, -43.2072) centre (125.5296, -43.2072) ccw
  arc A1447 (125.8346, -43.2072) -> (125.2246, -43.2072) centre (125.5296, -43.2072) ccw
  arc A1448 (155.4743, -39.6346) -> (156.0843, -39.6346) centre (155.7793, -39.6346) ccw
  arc A1449 (156.0843, -39.6346) -> (155.4743, -39.6346) centre (155.7793, -39.6346) ccw
  arc A1450 (182.3965, -14.2681) -> (183.0066, -14.2681) centre (182.7015, -14.2681) ccw
  arc A1451 (183.0066, -14.2681) -> (182.3965, -14.2681) centre (182.7015, -14.2681) ccw
  arc A1452 (131.6094, -30.2935) -> (132.2194, -30.2935) centre (131.9144, -30.2935) ccw
  arc A1453 (132.2194, -30.2935) -> (131.6094, -30.2935) centre (131.9144, -30.2935) ccw
  arc A1454 (16.2772, -59.686) -> (16.8872, -59.686) centre (16.5822, -59.686) ccw
  arc A1455 (16.8872, -59.686) -> (16.2772, -59.686) centre (16.5822, -59.686) ccw
  arc A1456 (214.4288, 38.2495) -> (215.0388, 38.2495) centre (214.7338, 38.2495) ccw
  arc A1457 (215.0388, 38.2495) -> (214.4288, 38.2495) centre (214.7338, 38.2495) ccw
  arc A1458 (15.3234, -1.528) -> (15.9334, -1.528) centre (15.6284, -1.528) ccw
  arc A1459 (15.9334, -1.528) -> (15.3234, -1.528) centre (15.6284, -1.528) ccw
  arc A1460 (133.3503, 19.914) -> (133.9603, 19.914) centre (133.6553, 19.914) ccw
  arc A1461 (133.9603, 19.914) -> (133.3503, 19.914) centre (133.6553, 19.914) ccw
  arc A1462 (38.3038, -41.9862) -> (38.9138, -41.9862) centre (38.6088, -41.9862) ccw
  arc A1463 (38.9138, -41.9862) -> (38.3038, -41.9862) centre (38.6088, -41.9862) ccw
  arc A1464 (95.9078, -39.4411) -> (96.5179, -39.4411) centre (96.2129, -39.4411) ccw
  arc A1465 (96.5179, -39.4411) -> (95.9078, -39.4411) centre (96.2129, -39.4411) ccw
  arc A1466 (151.4437, -40.1688) -> (150.8337, -40.1688) centre (151.1387, -40.1688) ccw
  arc A1467 (150.8337, -40.1688) -> (151.4437, -40.1688) centre (151.1387, -40.1688) ccw
  arc A1468 (44.5764, -41.9748) -> (45.1864, -41.9748) centre (44.8814, -41.9748) ccw
  arc A1469 (45.1864, -41.9748) -> (44.5764, -41.9748) centre (44.8814, -41.9748) ccw
  arc A1470 (163.8286, 37.8053) -> (164.4386, 37.8053) centre (164.1336, 37.8053) ccw
  arc A1471 (164.4386, 37.8053) -> (163.8286, 37.8053) centre (164.1336, 37.8053) ccw
  arc A1472 (145.9002, -13.2374) -> (146.5102, -13.2374) centre (146.2052, -13.2374) ccw
  arc A1473 (146.5102, -13.2374) -> (145.9002, -13.2374) centre (146.2052, -13.2374) ccw
  arc A1474 (176.2916, -9.8328) -> (176.9017, -9.8328) centre (176.5966, -9.8328) ccw
  arc A1475 (176.9017, -9.8328) -> (176.2916, -9.8328) centre (176.5966, -9.8328) ccw
  arc A1476 (115.7384, -12.0024) -> (116.3484, -12.0024) centre (116.0434, -12.0024) ccw
  arc A1477 (116.3484, -12.0024) -> (115.7384, -12.0024) centre (116.0434, -12.0024) ccw
  arc A1478 (150.9253, -10.1653) -> (150.3153, -10.1653) centre (150.6203, -10.1653) ccw
  arc A1479 (150.3153, -10.1653) -> (150.9253, -10.1653) centre (150.6203, -10.1653) ccw
  arc A1480 (85.8403, -12.5211) -> (86.4503, -12.5211) centre (86.1453, -12.5211) ccw
  arc A1481 (86.4503, -12.5211) -> (85.8403, -12.5211) centre (86.1453, -12.5211) ccw
  arc A1482 (117.0589, -9.5793) -> (116.4489, -9.5793) centre (116.7539, -9.5793) ccw
  arc A1483 (116.4489, -9.5793) -> (117.0589, -9.5793) centre (116.7539, -9.5793) ccw
  arc A1484 (43.7328, -19.9798) -> (44.3428, -19.9798) centre (44.0378, -19.9798) ccw
  arc A1485 (44.3428, -19.9798) -> (43.7328, -19.9798) centre (44.0378, -19.9798) ccw
  arc A1486 (91.481, -13.194) -> (90.871, -13.194) centre (91.176, -13.194) ccw
  arc A1487 (90.871, -13.194) -> (91.481, -13.194) centre (91.176, -13.194) ccw
  arc A1488 (217.1999, -62.0055) -> (217.81, -62.0055) centre (217.505, -62.0055) ccw
  arc A1489 (217.81, -62.0055) -> (217.1999, -62.0055) centre (217.505, -62.0055) ccw
  arc A1490 (186.3411, -6.5094) -> (185.7311, -6.5094) centre (186.0361, -6.5094) ccw
  arc A1491 (185.7311, -6.5094) -> (186.3411, -6.5094) centre (186.0361, -6.5094) ccw
  arc A1492 (150.7914, -28.8564) -> (150.1814, -28.8564) centre (150.4864, -28.8564) ccw
  arc A1493 (150.1814, -28.8564) -> (150.7914, -28.8564) centre (150.4864, -28.8564) ccw
  arc A1494 (145.5976, -60.2572) -> (144.9876, -60.2572) centre (145.2926, -60.2572) ccw
  arc A1495 (144.9876, -60.2572) -> (145.5976, -60.2572) centre (145.2926, -60.2572) ccw
  arc A1496 (120.0492, -66.7802) -> (119.4392, -66.7802) centre (119.7442, -66.7802) ccw
  arc A1497 (119.4392, -66.7802) -> (120.0492, -66.7802) centre (119.7442, -66.7802) ccw
  arc A1498 (168.0696, 11.5998) -> (168.6797, 11.5998) centre (168.3747, 11.5998) ccw
  arc A1499 (168.6797, 11.5998) -> (168.0696, 11.5998) centre (168.3747, 11.5998) ccw
  arc A1500 (194.5931, 20.9148) -> (195.2031, 20.9148) centre (194.8981, 20.9148) ccw
  arc A1501 (195.2031, 20.9148) -> (194.5931, 20.9148) centre (194.8981, 20.9148) ccw
  arc A1502 (99.482, 26.218) -> (98.872, 26.218) centre (99.177, 26.218) ccw
  arc A1503 (98.872, 26.218) -> (99.482, 26.218) centre (99.177, 26.218) ccw
  arc A1504 (70.5816, -16.6778) -> (69.9716, -16.6778) centre (70.2766, -16.6778) ccw
  arc A1505 (69.9716, -16.6778) -> (70.5816, -16.6778) centre (70.2766, -16.6778) ccw
  arc A1506 (134.7974, 16.8688) -> (135.4074, 16.8688) centre (135.1024, 16.8688) ccw
  arc A1507 (135.4074, 16.8688) -> (134.7974, 16.8688) centre (135.1024, 16.8688) ccw
  arc A1508 (165.3643, 20.1454) -> (165.9743, 20.1454) centre (165.6693, 20.1454) ccw
  arc A1509 (165.9743, 20.1454) -> (165.3643, 20.1454) centre (165.6693, 20.1454) ccw
  arc A1510 (100.7405, 26.9607) -> (101.3505, 26.9607) centre (101.0455, 26.9607) ccw
  arc A1511 (101.3505, 26.9607) -> (100.7405, 26.9607) centre (101.0455, 26.9607) ccw
  arc A1512 (87.1376, -6.1922) -> (86.5276, -6.1922) centre (86.8326, -6.1922) ccw
  arc A1513 (86.5276, -6.1922) -> (87.1376, -6.1922) centre (86.8326, -6.1922) ccw
  arc A1514 (104.8107, 16.8617) -> (104.2007, 16.8617) centre (104.5057, 16.8617) ccw
  arc A1515 (104.2007, 16.8617) -> (104.8107, 16.8617) centre (104.5057, 16.8617) ccw
  arc A1516 (124.9809, 15.4924) -> (124.3709, 15.4924) centre (124.6759, 15.4924) ccw
  arc A1517 (124.3709, 15.4924) -> (124.9809, 15.4924) centre (124.6759, 15.4924) ccw
  arc A1518 (20.6747, 14.645) -> (21.2847, 14.645) centre (20.9797, 14.645) ccw
  arc A1519 (21.2847, 14.645) -> (20.6747, 14.645) centre (20.9797, 14.645) ccw
  arc A1520 (21.6941, 18.769) -> (21.0841, 18.769) centre (21.3891, 18.769) ccw
  arc A1521 (21.0841, 18.769) -> (21.6941, 18.769) centre (21.3891, 18.769) ccw
  arc A1522 (38.4468, 16.8274) -> (39.0568, 16.8274) centre (38.7518, 16.8274) ccw
  arc A1523 (39.0568, 16.8274) -> (38.4468, 16.8274) centre (38.7518, 16.8274) ccw
  arc A1524 (75.5441, 20.0435) -> (76.1541, 20.0435) centre (75.8491, 20.0435) ccw
  arc A1525 (76.1541, 20.0435) -> (75.5441, 20.0435) centre (75.8491, 20.0435) ccw
  arc A1526 (217.0548, 36.5028) -> (216.4448, 36.5028) centre (216.7498, 36.5028) ccw
  arc A1527 (216.4448, 36.5028) -> (217.0548, 36.5028) centre (216.7498, 36.5028) ccw
  arc A1528 (62.906, 36.5028) -> (62.296, 36.5028) centre (62.601, 36.5028) ccw
  arc A1529 (62.296, 36.5028) -> (62.906, 36.5028) centre (62.601, 36.5028) ccw
  arc A1530 (124.3422, 49.6851) -> (124.9522, 49.6851) centre (124.6472, 49.6851) ccw
  arc A1531 (124.9522, 49.6851) -> (124.3422, 49.6851) centre (124.6472, 49.6851) ccw
  arc A1532 (93.4053, -27.5572) -> (92.7953, -27.5572) centre (93.1003, -27.5572) ccw
  arc A1533 (92.7953, -27.5572) -> (93.4053, -27.5572) centre (93.1003, -27.5572) ccw
  arc A1534 (158.7585, 44.4614) -> (159.3685, 44.4614) centre (159.0635, 44.4614) ccw
  arc A1535 (159.3685, 44.4614) -> (158.7585, 44.4614) centre (159.0635, 44.4614) ccw
  arc A1536 (184.6013, 44.4614) -> (185.2113, 44.4614) centre (184.9063, 44.4614) ccw
  arc A1537 (185.2113, 44.4614) -> (184.6013, 44.4614) centre (184.9063, 44.4614) ccw
  arc A1538 (118.5147, 12.5444) -> (119.1247, 12.5444) centre (118.8197, 12.5444) ccw
  arc A1539 (119.1247, 12.5444) -> (118.5147, 12.5444) centre (118.8197, 12.5444) ccw
  arc A1540 (127.6791, 57.1512) -> (127.0691, 57.1512) centre (127.3741, 57.1512) ccw
  arc A1541 (127.0691, 57.1512) -> (127.6791, 57.1512) centre (127.3741, 57.1512) ccw
  arc A1542 (129.448, 44.4614) -> (128.838, 44.4614) centre (129.143, 44.4614) ccw
  arc A1543 (128.838, 44.4614) -> (129.448, 44.4614) centre (129.143, 44.4614) ccw
  arc A1544 (159.8915, 50.1576) -> (159.2815, 50.1576) centre (159.5865, 50.1576) ccw
  arc A1545 (159.2815, 50.1576) -> (159.8915, 50.1576) centre (159.5865, 50.1576) ccw
  arc A1546 (98.789, 44.4614) -> (99.399, 44.4614) centre (99.094, 44.4614) ccw
  arc A1547 (99.399, 44.4614) -> (98.789, 44.4614) centre (99.094, 44.4614) ccw
  arc A1548 (107.27, 44.4614) -> (106.6599, 44.4614) centre (106.9649, 44.4614) ccw
  arc A1549 (106.6599, 44.4614) -> (107.27, 44.4614) centre (106.9649, 44.4614) ccw
  arc A1550 (113.4079, 50.5993) -> (112.7979, 50.5993) centre (113.1029, 50.5993) ccw
  arc A1551 (112.7979, 50.5993) -> (113.4079, 50.5993) centre (113.1029, 50.5993) ccw
  arc A1552 (129.6654, 50.5993) -> (129.0554, 50.5993) centre (129.3604, 50.5993) ccw
  arc A1553 (129.0554, 50.5993) -> (129.6654, 50.5993) centre (129.3604, 50.5993) ccw
  arc A1554 (69.3251, 44.4614) -> (68.7151, 44.4614) centre (69.0201, 44.4614) ccw
  arc A1555 (68.7151, 44.4614) -> (69.3251, 44.4614) centre (69.0201, 44.4614) ccw
  arc A1556 (100.1417, 49.9803) -> (99.5317, 49.9803) centre (99.8367, 49.9803) ccw
  arc A1557 (99.5317, 49.9803) -> (100.1417, 49.9803) centre (99.8367, 49.9803) ccw
  arc A1558 (51.4892, 50.5033) -> (50.8791, 50.5033) centre (51.1842, 50.5033) ccw
  arc A1559 (50.8791, 50.5033) -> (51.4892, 50.5033) centre (51.1842, 50.5033) ccw
  arc A1560 (73.958, 49.883) -> (73.348, 49.883) centre (73.653, 49.883) ccw
  arc A1561 (73.348, 49.883) -> (73.958, 49.883) centre (73.653, 49.883) ccw
  arc A1562 (220.95, -27.0019) -> (221.56, -27.0019) centre (221.255, -27.0019) ccw
  arc A1563 (221.56, -27.0019) -> (220.95, -27.0019) centre (221.255, -27.0019) ccw
  arc A1564 (218.0011, 60.5599) -> (218.6111, 60.5599) centre (218.3061, 60.5599) ccw
  arc A1565 (218.6111, 60.5599) -> (218.0011, 60.5599) centre (218.3061, 60.5599) ccw
  arc A1566 (44.1071, 60.5599) -> (43.4971, 60.5599) centre (43.8021, 60.5599) ccw
  arc A1567 (43.4971, 60.5599) -> (44.1071, 60.5599) centre (43.8021, 60.5599) ccw
  arc A1568 (189.306, 74.8421) -> (188.696, 74.8421) centre (189.001, 74.8421) ccw
  arc A1569 (188.696, 74.8421) -> (189.306, 74.8421) centre (189.001, 74.8421) ccw
  arc A1570 (201.3944, 74.8421) -> (200.7844, 74.8421) centre (201.0894, 74.8421) ccw
  arc A1571 (200.7844, 74.8421) -> (201.3944, 74.8421) centre (201.0894, 74.8421) ccw
  arc A1572 (95.6812, 66.3102) -> (95.0712, 66.3102) centre (95.3762, 66.3102) ccw
  arc A1573 (95.0712, 66.3102) -> (95.6812, 66.3102) centre (95.3762, 66.3102) ccw
  arc A1574 (64.4041, -23.0278) -> (63.7941, -23.0278) centre (64.0991, -23.0278) ccw
  arc A1575 (63.7941, -23.0278) -> (64.4041, -23.0278) centre (64.0991, -23.0278) ccw
  arc A1576 (92.477, -20.5656) -> (91.867, -20.5656) centre (92.172, -20.5656) ccw
  arc A1577 (91.867, -20.5656) -> (92.477, -20.5656) centre (92.172, -20.5656) ccw
  arc A1578 (65.9685, 83.9028) -> (65.3584, 83.9028) centre (65.6634, 83.9028) ccw
  arc A1579 (65.3584, 83.9028) -> (65.9685, 83.9028) centre (65.6634, 83.9028) ccw
  arc A1580 (35.3066, -9.865) -> (35.9166, -9.865) centre (35.6116, -9.865) ccw
  arc A1581 (35.9166, -9.865) -> (35.3066, -9.865) centre (35.6116, -9.865) ccw
  arc A1582 (35.9144, -3.5704) -> (35.3043, -3.5704) centre (35.6093, -3.5704) ccw
  arc A1583 (35.3043, -3.5704) -> (35.9144, -3.5704) centre (35.6093, -3.5704) ccw
  arc A1584 (68.952, 74.231) -> (69.5621, 74.231) centre (69.257, 74.231) ccw
  arc A1585 (69.5621, 74.231) -> (68.952, 74.231) centre (69.257, 74.231) ccw
  arc A1586 (104.4557, 74.231) -> (105.0657, 74.231) centre (104.7607, 74.231) ccw
  arc A1587 (105.0657, 74.231) -> (104.4557, 74.231) centre (104.7607, 74.231) ccw
  arc A1588 (18.3112, -49.6804) -> (18.9212, -49.6804) centre (18.6162, -49.6804) ccw
  arc A1589 (18.9212, -49.6804) -> (18.3112, -49.6804) centre (18.6162, -49.6804) ccw
  arc A1590 (22.2287, -60.4264) -> (22.8387, -60.4264) centre (22.5337, -60.4264) ccw
  arc A1591 (22.8387, -60.4264) -> (22.2287, -60.4264) centre (22.5337, -60.4264) ccw
  arc A1592 (142.1906, 77.1248) -> (142.8006, 77.1248) centre (142.4956, 77.1248) ccw
  arc A1593 (142.8006, 77.1248) -> (142.1906, 77.1248) centre (142.4956, 77.1248) ccw
  arc A1594 (134.2777, 77.1248) -> (134.8877, 77.1248) centre (134.5827, 77.1248) ccw
  arc A1595 (134.8877, 77.1248) -> (134.2777, 77.1248) centre (134.5827, 77.1248) ccw
  arc A1596 (155.317, 57.7646) -> (155.9271, 57.7646) centre (155.622, 57.7646) ccw
  arc A1597 (155.9271, 57.7646) -> (155.317, 57.7646) centre (155.622, 57.7646) ccw
  arc A1598 (159.4329, 57.7646) -> (160.0429, 57.7646) centre (159.7379, 57.7646) ccw
  arc A1599 (160.0429, 57.7646) -> (159.4329, 57.7646) centre (159.7379, 57.7646) ccw
  arc A1600 (5.8887, 29.8711) -> (5.2787, 29.8711) centre (5.5837, 29.8711) ccw
  arc A1601 (5.2787, 29.8711) -> (5.8887, 29.8711) centre (5.5837, 29.8711) ccw
  arc A1602 (13.3844, -37.0289) -> (13.9944, -37.0289) centre (13.6894, -37.0289) ccw
  arc A1603 (13.9944, -37.0289) -> (13.3844, -37.0289) centre (13.6894, -37.0289) ccw
  arc A1604 (13.2263, -57.8284) -> (12.6163, -57.8284) centre (12.9213, -57.8284) ccw
  arc A1605 (12.6163, -57.8284) -> (13.2263, -57.8284) centre (12.9213, -57.8284) ccw
  arc A1606 (16.3452, -57.3339) -> (16.9552, -57.3339) centre (16.6502, -57.3339) ccw
  arc A1607 (16.9552, -57.3339) -> (16.3452, -57.3339) centre (16.6502, -57.3339) ccw
  arc A1608 (10.7886, 67.0153) -> (10.1786, 67.0153) centre (10.4836, 67.0153) ccw
  arc A1609 (10.1786, 67.0153) -> (10.7886, 67.0153) centre (10.4836, 67.0153) ccw
  arc A1610 (14.3196, 16.4842) -> (14.9296, 16.4842) centre (14.6246, 16.4842) ccw
  arc A1611 (14.9296, 16.4842) -> (14.3196, 16.4842) centre (14.6246, 16.4842) ccw
  arc A1612 (23.1215, 16.4842) -> (23.7315, 16.4842) centre (23.4265, 16.4842) ccw
  arc A1613 (23.7315, 16.4842) -> (23.1215, 16.4842) centre (23.4265, 16.4842) ccw
  arc A1614 (16.6645, -56.3786) -> (17.2745, -56.3786) centre (16.9695, -56.3786) ccw
  arc A1615 (17.2745, -56.3786) -> (16.6645, -56.3786) centre (16.9695, -56.3786) ccw
  arc A1616 (14.7125, -53.6621) -> (15.3225, -53.6621) centre (15.0175, -53.6621) ccw
  arc A1617 (15.3225, -53.6621) -> (14.7125, -53.6621) centre (15.0175, -53.6621) ccw
  arc A1618 (15.7661, -61.0169) -> (16.3761, -61.0169) centre (16.0711, -61.0169) ccw
  arc A1619 (16.3761, -61.0169) -> (15.7661, -61.0169) centre (16.0711, -61.0169) ccw
  arc A1620 (160.9081, -5.432) -> (161.5181, -5.432) centre (161.2131, -5.432) ccw
  arc A1621 (161.5181, -5.432) -> (160.9081, -5.432) centre (161.2131, -5.432) ccw
  arc A1622 (41.8068, -4.8617) -> (42.4168, -4.8617) centre (42.1118, -4.8617) ccw
  arc A1623 (42.4168, -4.8617) -> (41.8068, -4.8617) centre (42.1118, -4.8617) ccw
  arc A1624 (217.5622, 48.9513) -> (218.1722, 48.9513) centre (217.8672, 48.9513) ccw
  arc A1625 (218.1722, 48.9513) -> (217.5622, 48.9513) centre (217.8672, 48.9513) ccw
  arc A1626 (193.146, -2.8919) -> (192.536, -2.8919) centre (192.841, -2.8919) ccw
  arc A1627 (192.536, -2.8919) -> (193.146, -2.8919) centre (192.841, -2.8919) ccw
  arc A1628 (208.5449, 31.9866) -> (209.1549, 31.9866) centre (208.8499, 31.9866) ccw
  arc A1629 (209.1549, 31.9866) -> (208.5449, 31.9866) centre (208.8499, 31.9866) ccw
  arc A1630 (186.3153, 14.4761) -> (186.9253, 14.4761) centre (186.6203, 14.4761) ccw
  arc A1631 (186.9253, 14.4761) -> (186.3153, 14.4761) centre (186.6203, 14.4761) ccw
  arc A1632 (195.1222, 7.3252) -> (195.7322, 7.3252) centre (195.4272, 7.3252) ccw
  arc A1633 (195.7322, 7.3252) -> (195.1222, 7.3252) centre (195.4272, 7.3252) ccw
  arc A1634 (12.759, -60.0847) -> (13.369, -60.0847) centre (13.064, -60.0847) ccw
  arc A1635 (13.369, -60.0847) -> (12.759, -60.0847) centre (13.064, -60.0847) ccw
  arc A1636 (10.9078, 12.8002) -> (11.5179, 12.8002) centre (11.2129, 12.8002) ccw
  arc A1637 (11.5179, 12.8002) -> (10.9078, 12.8002) centre (11.2129, 12.8002) ccw
  arc A1638 (9.2652, 70.1903) -> (9.8752, 70.1903) centre (9.5702, 70.1903) ccw
  arc A1639 (9.8752, 70.1903) -> (9.2652, 70.1903) centre (9.5702, 70.1903) ccw
  arc A1640 (187.8959, 15.9968) -> (188.5059, 15.9968) centre (188.2009, 15.9968) ccw